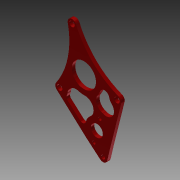
# Autodesk Inventor part: OutlineSketch1
Saved by Autodesk Inventor 2013 (Build 170138000, 138)
## iProperties
Created: 2013-06-03
Part Number: OutlineSketch1
Material: Aluminum 6061
Document SubType Name: Modeling
Designer: mvarma
Density: 1 g/cm^3
Author: mvarma
Autodesk Inventor part; units mm, degrees
ref_plane "YZ Plane" through (0, 0, 0) normal (1, 0, 0) x (0, 1, 0)
ref_plane "XZ Plane" through (0, 0, 0) normal (0, 1, 0) x (-1, 0, 0)
ref_plane "XY Plane" through (0, 0, 0) normal (0, 0, 1) x (1, 0, 0)
sketch "Sketch1" plane through (0, 0, 0) normal (0, 0, 1) x (1, 0, 0)
  line L0 (0, 0) -> (304.8, 0) construction
  line L1 (304.8, 0) -> (304.8, 50.8) construction
  line L2 (304.8, 50.8) -> (0, 50.8) construction
  line L3 (0, 50.8) -> (0, 0) construction
  circle A0 centre (152.4, 22.225) radius 6.35 construction
  circle A1 centre (152.4, 22.225) radius 34.29 construction
  circle A2 centre (152.4, 22.225) radius 22.225 construction
  line L4 (152.4, 22.225) -> (140.5275, 60.4809) construction
  circle A3 centre (140.5275, 60.4809) radius 9.525 construction
  circle A4 centre (140.5275, 60.4809) radius 17.78 construction
  circle A5 centre (93.2037, 85.09) radius 31.75 construction
  circle A6 centre (165.6038, 107.5589) radius 31.75 construction
  circle A7 centre (223.2898, 85.09) radius 31.75 construction
  line L5 (0, 50.8) -> (0, 53.34) construction
  line L6 (0, 53.34) -> (304.8, 53.34) construction
  line L7 (304.8, 53.34) -> (304.8, 50.8) construction
  circle A8 centre (140.5275, 60.4809) radius 21.59 construction
  circle A9 centre (152.4, 22.225) radius 46.99 construction
  circle A10 centre (152.4, 22.225) radius 50.8 construction
  arc A11 (87.8811, 79.5952) -> (94.2788, 92.6641) centre (93.2037, 85.09) ccw construction
  circle A12 centre (165.6038, 107.5589) radius 7.65 construction
  arc A13 (222.7819, 92.7231) -> (227.035, 78.4195) centre (223.2898, 85.09) ccw construction
  circle A14 centre (165.6038, 107.5589) radius 9.1 construction
  circle A15 centre (140.5275, 60.4809) radius 22.9 construction
  line L8 (87.8811, 79.5952) -> (124.5946, 44.0324) construction
  line L9 (173.1021, 106.043) -> (162.9734, 55.943) construction
  line L10 (94.2788, 92.6641) -> (93.2037, 85.09) construction
  line L11 (93.2037, 85.09) -> (87.8811, 79.5952) construction
  circle A16 centre (129.608, 95.6662) radius 3.9688
  circle A17 centre (129.608, 95.6662) radius 7.9375 construction
  line L12 (94.2788, 92.6641) -> (128.4925, 87.8075) construction
  line L13 (134.9768, 89.8198) -> (160.4294, 113.1935) construction
  line L14 (160.4294, 113.1935) -> (165.6038, 107.5589) construction
  line L15 (173.1021, 106.043) -> (165.6038, 107.5589) construction
  line L16 (140.5275, 60.4809) -> (129.608, 95.6662) construction
  line L17 (93.2037, 85.09) -> (165.6038, 107.5589) construction
  line L18 (152.4, 22.225) -> (93.2037, 85.09) construction
  line L19 (152.4, 22.225) -> (165.6038, 107.5589) construction
  circle A18 centre (129.608, 95.6662) radius 9.2075 construction
  circle A19 centre (129.608, 95.6662) radius 6.1595 construction
  arc A20 (94.2788, 92.6641) -> (87.8811, 79.5952) centre (93.2037, 85.09) ccw construction
  circle A21 centre (165.6038, 107.5589) radius 25.4 construction
  circle A22 centre (223.2898, 85.09) radius 25.4 construction
  line L20 (107.1636, 113.6064) -> (79.2438, 56.5736) construction
  circle A23 centre (93.2037, 85.09) radius 25.4 construction
  line L21 (214.2406, 115.5231) -> (232.339, 54.6569) construction
  line L22 (57.6437, 183.7589) -> (210.0437, 183.7589)
  line L23 (210.0437, 183.7589) -> (210.0437, -6.7411)
  line L24 (210.0437, -6.7411) -> (57.6437, -6.7411)
  line L25 (57.6437, -6.7411) -> (57.6437, 183.7589)
  circle A24 centre (140.5275, 60.4809) radius 11.1125
  arc A25 (226.9198, 75.5499) -> (222.1074, 95.2918) centre (224.5136, 85.4209) ccw construction
  line L26 (222.084, 84.6985) -> (230.5292, 60.7435) construction
  line L27 (224.5136, 85.4209) -> (230.5292, 60.7435) construction
  line L28 (222.084, 84.6985) -> (213.6389, 108.6534) construction
  line L29 (224.5136, 85.4209) -> (218.498, 110.0983) construction
  arc A26 (212.8472, 110.8992) -> (214.4306, 106.4076) centre (213.6389, 108.6534) ccw construction
  arc A27 (219.062, 107.7848) -> (217.9341, 112.4118) centre (218.498, 110.0983) ccw construction
  arc A28 (219.062, 107.7848) -> (214.4306, 106.4076) centre (230.5292, 60.7435) ccw construction
  arc A29 (217.9341, 112.4118) -> (212.8472, 110.8992) centre (230.5292, 60.7435) ccw construction
  line L30 (213.6389, 108.6534) -> (212.8472, 110.8992) construction
  line L31 (218.498, 110.0983) -> (217.9341, 112.4118) construction
  arc A30 (222.1074, 95.2918) -> (218.706, 94.2804) centre (230.5292, 60.7435) ccw construction
  arc A31 (226.9198, 75.5499) -> (225.4621, 75.1165) centre (230.5292, 60.7435) ccw construction
  line L32 (106.6203, 106.7318) -> (94.3281, 84.5044) construction
  line L33 (82.0358, 62.2769) -> (92.0515, 85.6188) construction
  arc A32 (103.0062, 111.1491) -> (101.1282, 106.7724) centre (102.0672, 108.9607) ccw construction
  arc A33 (105.4679, 104.648) -> (107.7727, 108.8157) centre (106.6203, 106.7318) ccw construction
  arc A34 (105.4679, 104.648) -> (101.1282, 106.7724) centre (82.0358, 62.2769) ccw construction
  line L34 (102.0672, 108.9607) -> (103.0062, 111.1491) construction
  line L35 (106.6203, 106.7318) -> (107.7727, 108.8157) construction
  arc A35 (107.7727, 108.8157) -> (103.0062, 111.1491) centre (82.0358, 62.2769) ccw construction
  arc A36 (218.706, 94.2804) -> (225.4621, 75.1165) centre (222.084, 84.6985) ccw construction
  arc A37 (89.4112, 75.6134) -> (99.245, 93.3953) centre (94.3281, 84.5044) ccw construction
  line L36 (92.0515, 85.6188) -> (102.0672, 108.9607) construction
  line L37 (94.3281, 84.5044) -> (82.0358, 62.2769) construction
  arc A38 (89.4112, 75.6134) -> (88.0452, 76.282) centre (82.0358, 62.2769) ccw construction
  arc A39 (99.245, 93.3953) -> (96.0578, 94.9556) centre (82.0358, 62.2769) ccw construction
  arc A40 (96.0578, 94.9556) -> (88.0452, 76.282) centre (92.0515, 85.6188) ccw construction
  line L38 (165.6038, 107.5589) -> (143.4823, 120.0409) construction
  line L39 (165.6038, 107.5589) -> (187.7253, 95.0769) construction
  circle A41 centre (140.5275, 60.4809) radius 26.71 construction
  line L40 (222.7819, 92.7231) -> (138.7542, 87.1319) construction
  line L41 (227.035, 78.4195) -> (153.6041, 37.1908) construction
  line L42 (223.2898, 85.09) -> (222.7819, 92.7231) construction
  line L43 (223.2898, 85.09) -> (227.035, 78.4195) construction
  line L44 (140.5275, 60.4809) -> (138.7542, 87.1319) construction
  line L45 (140.5275, 60.4809) -> (153.6041, 37.1908) construction
  arc A42 (227.035, 78.4195) -> (222.7819, 92.7231) centre (223.2898, 85.09) ccw construction
  arc A43 (227.035, 78.4195) -> (226.3078, 78.0605) centre (223.2898, 85.09) ccw construction
  line L46 (140.5275, 60.4809) -> (223.2898, 85.09) construction
  circle A44 centre (140.5275, 60.4809) radius 15.875
  circle A45 centre (118.222, 39.4179) radius 3.9688
  circle A46 centre (170.8389, 55.7472) radius 3.9688
  circle A47 centre (57.8579, 80.9136) radius 69.2823
  circle A48 centre (197.1037, 124.1276) radius 69.2823
  arc A49 (163.3226, 13.1136) -> (164.7609, 15.1872) centre (152.4, 22.225) ccw
  circle A50 centre (152.4, 22.225) radius 11.176 construction
  circle A51 centre (152.4, 22.225) radius 19.05 construction
  line L47 (115.5534, 36.4803) -> (142.8358, 11.6966)
  line L48 (152.4, 22.225) -> (142.8358, 11.6966) construction
  line L49 (174.7018, 54.8366) -> (166.2445, 18.9613) construction
  line L50 (152.4, 22.225) -> (166.2445, 18.9613) construction
  arc A52 (154.1883, 3.1005) -> (155.4853, 0.9992) centre (158.0464, 4.031) ccw
  line L51 (152.4, 22.225) -> (158.0464, 4.031) construction
  arc A53 (156.616, 8.6402) -> (163.3226, 13.1136) centre (152.4, 22.225) ccw
  arc A54 (150.0325, 8.1994) -> (156.616, 8.6402) centre (152.4, 22.225) ccw
  arc A55 (156.8701, 7.8214) -> (154.1883, 3.1005) centre (158.0464, 4.031) ccw
  arc A56 (161.5818, 5.8343) -> (156.8701, 7.8214) centre (158.0464, 4.031) ccw
  line L52 (143.2212, 11.3589) -> (155.4853, 0.9992)
  line L53 (161.8739, 2.9818) -> (166.118, 18.4648) construction
  line L54 (143.2212, 11.3589) -> (152.4, 22.225) construction
  line L55 (152.4, 22.225) -> (166.118, 18.4648) construction
  arc A57 (166.118, 18.4648) -> (166.2445, 18.9613) centre (152.4, 22.225) ccw
  arc A58 (166.2445, 18.9613) -> (166.6216, 22.4887) centre (152.4, 22.225) ccw construction
  arc A59 (142.8358, 11.6966) -> (143.2212, 11.3589) centre (152.4, 22.225) ccw
  arc A60 (143.2212, 11.3589) -> (150.0325, 8.1994) centre (152.4, 22.225) ccw
  circle A61 centre (152.4, 22.225) radius 5.5065
  line L56 (152.4, 22.225) -> (166.1835, 18.7125)
  line L57 (166.6216, 22.4887) -> (164.7609, 15.1872)
  arc A62 (164.7609, 15.1872) -> (166.118, 18.4648) centre (152.4, 22.225) ccw construction
  line L58 (164.7609, 15.1872) -> (161.9087, 3.1183)
  line L59 (158.0464, 4.031) -> (161.9087, 3.1183) construction
  arc A63 (166.6216, 22.4887) -> (142.8358, 11.6966) centre (152.4, 22.225) ccw
  line L60 (170.8389, 55.7472) -> (174.6893, 54.7854) construction
  line L61 (174.6893, 54.7854) -> (166.6216, 22.4887)
  line L62 (155.1599, 33.0549) -> (149.6401, 11.3951) construction
  circle A64 centre (155.1599, 33.0549) radius 2.1082
  circle A65 centre (149.6401, 11.3951) radius 2.1082
  arc A66 (161.9087, 3.1183) -> (161.5818, 5.8343) centre (158.0464, 4.031) ccw
  arc A67 (155.4853, 0.9992) -> (161.9087, 3.1183) centre (158.0464, 4.031) ccw
  point P0 (216.0504, 109.4365)
  point P1 (104.3716, 107.9031)
  point P2 (146.0332, 45.5912)
  point P3 (172.2619, 59.4521)
  point P4 (114.9515, 41.6662)
  point P5 (133.2649, 97.2082)
  point P6 (125.7206, 94.8669)
  dimension "d127" = 31.75
  dimension "d150" = 38.1
  dimension "d1" = 50.8
  dimension "d3" = 22.225
  dimension "d4" = 152.4
  dimension "d7" = 68.58
  dimension "d8" = 44.45
  dimension "d9" = 19.05
  dimension "d10" = 35.56
  dimension "d11" = 40.0558
  dimension "d12" = 63.5
  dimension "d13" = 63.5
  dimension "d14" = 63.5
  dimension "d15" = 2.54
  dimension "d16" = 304.8
  dimension "d17" = 43.18
  dimension "d18" = 93.98
  dimension "d19" = 101.6
  dimension "d21" = 15.3
  dimension "d22" = 15.3
  dimension "d24" = 18.2
  dimension "d29" = 45.8
  dimension "d30" = 143.991
  dimension "d31" = 7.9375
  dimension "d32" = 15.875
  dimension "d33" = 143.991
  dimension "d35" = 18.415
  dimension "d37" = 12.319
  dimension "d40" = 50.8
  dimension "d41" = 50.8
  dimension "d42" = 18.004
  dimension "d43" = 18.004
  dimension "d44" = 50.8
  dimension "d53" = 152.4
  dimension "d54" = 190.5
  dimension "d55" = 35.56
  dimension "d56" = 76.2
  dimension "d57" = 22.225
  dimension "d67" = 25.4
  dimension "d68" = 25.4
  dimension "d69" = 2.86
  dimension "d70" = 25.4
  dimension "d71" = 25.4
  dimension "d72" = 4.7625
  dimension "d75" = 2.86
  dimension "d80" = 4.7625
  dimension "d82" = 4.7625
  dimension "d83" = 50.8
  dimension "d84" = 50.8
  dimension "d85" = 10.16
  dimension "d97" = 48.4188
  dimension "d99" = 20.32
  dimension "d101" = 25.4
  dimension "d102" = 25.4
  dimension "d103" = 10.16
  dimension "d105" = 18.004
  dimension "d106" = 18.004
  dimension "d107" = 53.42
  dimension "d108" = 154.494
  dimension "d109" = 7.65
  dimension "d111" = 86.3435
  dimension "d112" = 12.753
  dimension "d113" = 12.753
  dimension "d135" = 7.9375
  dimension "d136" = 7.9375
  dimension "d149" = 22.352
  constraints: 130 end point, 112 point on circle, 66 centre point, 56 tangent, 41 coincident, 16 point on line, 14 perpendicular, 10 collinear, 8 parallel, 3 midpoint, 2 horizontal, 1 equal radius, 11 other
  measures "d1" distance of L1.end L0.end
  measures "d3" distance from line of L0 A0.centre
  measures "d4" distance from line of L3 A0.centre
  measures "d7" diameter of A1
  measures "d8" diameter of A2
  measures "d9" diameter of A3
  measures "d10" diameter of A4
  measures "d11" distance of L4.start L4.end
  measures "d12" diameter of A5
  measures "d13" diameter of A6
  measures "d14" diameter of A7
  measures "d15" distance of L2.end L5.end
  measures "d16" distance of L0.end L0.start
  measures "d17" diameter of A8
  measures "d18" diameter of A9
  measures "d19" diameter of A10
  measures "d21" diameter of A11
  measures "d22" diameter of A12
  measures "d24" diameter of A14
  measures "d29" diameter of A15
  measures "d30" angle of L11 L10
  measures "d31" diameter of A16
  measures "d32" diameter of A17
  measures "d33" angle of L15 L14
  measures "d35" diameter of A18
  measures "d37" diameter of A19
  measures "d40" diameter of A21
  measures "d41" diameter of A22
  measures "d42" angle of L10 L20
  measures "d43" angle of L11 L20
  measures "d44" diameter of A23
  measures "d53" distance of L23.end L24.end
  measures "d54" distance of L22.end L23.end
  measures "d55" distance from line of L25 A5.centre
  measures "d56" distance from line of L22 A6.centre
  measures "d57" diameter of A24
  measures "d67" distance of L26.start L26.end
  measures "d68" distance of L27.start L26.end
  measures "d69" angle of L21 L26
  measures "d70" distance of L26.start L28.end
  measures "d71" distance of L27.start L29.end
  measures "d72" diameter of A26
  measures "d75" angle of L20 L32
  measures "d80" diameter of A32
  measures "d82" diameter of A33
  measures "d83" distance of L33.start L36.end
  measures "d84" distance of L32.start L33.start
  measures "d85" radius of A25
  measures "d97" radius of A34
  measures "d99" diameter of A37
  measures "d101" distance of L33.start L33.end
  measures "d102" distance of L32.end L33.start
  measures "d103" radius of A40
  measures "d105" angle of L38 L14
  measures "d106" angle of L39 L15
  measures "d107" diameter of A41
  measures "d108" angle of L42 L43
  measures "d109" radius of A13
  measures "d111" distance of L44.start L42.start
  measures "d112" angle of L21 L42
  measures "d113" angle of L21 L43
  measures "d135" diameter of A45
  measures "d136" diameter of A46
  measures "d149" diameter of A50
extrude "Extrusion3" add sketch "Sketch1" along normal blind 3.175 contours A16 | A16 A48 A44 A47 | A48 A46 L61 A63 L47 A45 A47 A44 | A44 | A46 | A45 | L57 A49 A53 A54 A60 A59 A63 | A60 A54 A53 A49 L58 A66 A56 A55 A52 L52 | A52 A55 A56 A66 A67 | A64 | A65
hole "Hole3" at (82.0358, 62.2769, 0) at (230.5292, 60.7435, 0) at (187.7253, 95.0769, 0) at (216.0504, 109.4365, 0) at (118.222, 39.4179, 0) at (170.8389, 55.7472, 0) at (129.608, 95.6662, 0) direction (0, 0, 1) diameter 4.9784 end through all clearance for "Socket Head Cap Screw" size "#10" standard "Ansi Unified Screw Threads"
hole "Hole4" at (103.0062, 111.1491, 0) at (107.7727, 108.8157, 0) at (143.4823, 120.0409, 0) at (104.3716, 107.9031, 0) at (158.0464, 4.031, 0) direction (0, 0, 1) diameter 3.6576 end through all clearance for "Flat Head Machine Screw (82)" size "#6" standard "Ansi Unified Screw Threads"
hole "Hole5" at (155.1599, 33.0549, 0) at (149.6401, 11.3951, 0) direction (0, 0, 1) diameter 2.9464 end through all clearance for "Socket Head Cap Screw" size "#4" standard "Ansi Unified Screw Threads"
fillet "Fillet2" radius 3.175 2 edges at (164.7609, 15.1872, 1.5875) (166.6216, 22.4887, 1.5875)
sketch "Sketch3" plane through (0, 0, 3.175) normal (0, 0, 1) x (1, 0, 0)
  circle A0 centre (152.4, 22.225) radius 5.5065 projected
  circle A1 centre (140.5275, 60.4809) radius 11.1125 projected
  circle A2 centre (118.222, 39.4179) radius 2.4892 projected
  circle A3 centre (149.6401, 11.3951) radius 1.4732 projected
  circle A4 centre (155.1599, 33.0549) radius 1.4732 projected
  arc A5 (142.3415, 24.2936) -> (146.2577, 30.4544) centre (152.4, 22.225) ccw
  circle A6 centre (155.1599, 33.0549) radius 6.2357
  arc A7 (125.4359, 38.6786) -> (124.8466, 36.4681) centre (118.222, 39.4179) ccw
  arc A8 (141.2121, 44.6206) -> (135.6704, 45.3672) centre (140.5275, 60.4809) ccw
  arc A9 (125.4359, 38.6786) -> (135.6704, 45.3672) centre (133.263, 37.8764) ccw construction
  arc A10 (141.2121, 44.6206) -> (146.2577, 30.4544) centre (141.5514, 36.7598) ccw construction
  line L0 (118.222, 39.4179) -> (125.6337, 32.8072)
  arc A11 (125.6337, 32.8072) -> (124.8466, 36.4681) centre (127.7471, 35.1766) ccw construction
  arc A12 (137.1182, 22.5638) -> (142.3415, 24.2936) centre (139.2316, 24.9332) ccw
  arc A13 (124.8466, 36.4681) -> (125.6337, 32.8072) centre (127.7471, 35.1766) ccw
  arc A14 (135.6704, 45.3672) -> (125.4359, 38.6786) centre (133.263, 37.8764) ccw
  arc A15 (124.8466, 36.4681) -> (125.4359, 38.6786) centre (118.222, 39.4179) ccw
  arc A16 (135.6704, 45.3672) -> (141.2121, 44.6206) centre (140.5275, 60.4809) ccw
  arc A17 (149.1432, 34.6929) -> (141.2121, 44.6206) centre (141.5514, 36.7598) ccw
  arc A18 (146.2577, 30.4544) -> (149.1432, 34.6929) centre (141.5514, 36.7598) ccw
  arc A19 (146.2577, 30.4544) -> (142.3415, 24.2936) centre (152.4, 22.225) ccw
  arc A20 (142.3415, 24.2936) -> (137.1182, 22.5638) centre (139.2316, 24.9332) ccw construction
  line L1 (137.1182, 22.5638) -> (149.6401, 11.3951)
  line L2 (125.6337, 32.8072) -> (137.1182, 22.5638)
  line L3 (166.6234, 22.4959) -> (174.6893, 54.7854) projected
  arc A21 (133.2649, 97.2082) -> (172.2619, 59.4521) centre (197.1037, 124.1276) ccw projected
  circle A22 centre (170.8389, 55.7472) radius 2.4892 projected
  arc A23 (153.2986, 51.0513) -> (157.127, 38.9722) centre (159.5966, 46.4012) ccw
  arc A24 (157.127, 38.9722) -> (153.2986, 51.0513) centre (159.5966, 46.4012) ccw construction
  circle A25 centre (170.8389, 55.7472) radius 7.2517
  arc A26 (155.4506, 55.0663) -> (163.7136, 54.3993) centre (159.4907, 53.6004) ccw construction
  arc A27 (163.7136, 54.3993) -> (155.4506, 55.0663) centre (159.4907, 53.6004) ccw
  arc A28 (165.8729, 50.4627) -> (157.8357, 38.6873) centre (160.9319, 45.2046) ccw construction
  line L4 (168.7317, 46.6568) -> (166.5424, 37.8926) construction
  arc A29 (166.864, 49.312) -> (165.8729, 50.4627) centre (160.9319, 45.2046) ccw
  arc A30 (157.8357, 38.6873) -> (166.864, 49.312) centre (160.9319, 45.2046) ccw
  point P0 (0, 0)
  dimension "d194" = 4.7625
  dimension "d195" = 4.7625
  dimension "d196" = 4.7625
  dimension "d197" = 4.7625
  dimension "d200" = 6.35
  dimension "d201" = 6.35
  dimension "d204" = 4.7625
  dimension "d205" = 4.7625
  dimension "d206" = 6.35
  dimension "d208" = 3.81
  constraints: 52 point on circle, 24 centre point, 21 tangent, 8 end point, 5 coincident, 1 equal radius, 1 parallel
  measures "d194" radial gap between concentric circles of A2 A7
  measures "d195" radial gap between concentric circles of A4 A6
  measures "d196" radial gap between concentric circles of A0 A5
  measures "d197" radial gap between concentric circles of A1 A8
  measures "d200" diameter of A11
  measures "d201" diameter of A12
  measures "d205" radial gap between concentric circles of A22 A25
  measures "d208" distance between parallel lines of L3 L4
extrude "Extrusion5" cut sketch "Sketch3" against normal through all contours A19 A12 L2 A13 A15 A14 A16 A17 A18 | A6 A23 A8 A27 A25 A29 A30
equation "\"d8\" = Gear35tPD"
equation "\"d9\" = Gear15tPD"
equation "\"d10\" = Gear28tPD"
equation "\"d11\" = 0.5 * Gear48tPD + 0.5 * Gear15tPD + MeshingClearance"
equation "\"d12\" = CimOD"
equation "\"d13\" = CimOD"
equation "\"d14\" = CimOD"
equation "\"d17\" = Gear28tPD + ClearanceDiameter"
equation "\"d18\" = WheelOD"
equation "\"d19\" = WheelClearance"
equation "\"Pulley48tPD\" = 45.8"
equation "\"Pulley19tPD\" = 18.2"
equation "\"Pulley16tPD\" = 15.3"
equation "\"Gear15tPD\" = 19.05"
equation "\"Gear35tPD\" = 44.45"
equation "\"Gear48tPD\" = 60.96"
equation "\"Gear28tPD\" = 35.56"
equation "\"BearingLargeOD\" = 28.575"
equation "\"BearingSmallOD\" = 22.225"
equation "\"MeshingClearance\" = 0.0508"
equation "\"CimOD\" = 63.5"
equation "\"WheelOD\" = 93.98"
equation "\"ClearanceDiameter\" = 7.62"
equation "\"WheelClearance\" = 101.6"
equation "\"TensioningBearingID\" = 6.35"
equation "\"TensioningBearingOD\" = 15.875"
equation "\"SpingClipClearance\" = 8.89"
equation "\"Pi\" = 79.79645"
equation "\"Pulley56tPD\" = 53.5"
equation "\"BearingXLargeOD\" = 34.925"
body "Solid3"
